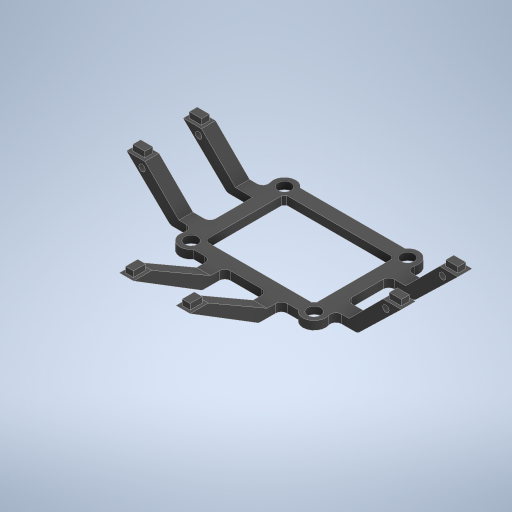
# Autodesk Inventor part: BasePlate
Saved by Autodesk Inventor 2024.2 (Build 282272000, 272)
## iProperties
Created: 2024-04-02
Part Number: BasePlate
Material: Generic
Document SubType Name: Modeling
Designer: ringl
Density: 1 g/cm^3
Appearance: Default(1)
Author: ringl
Autodesk Inventor part; units mm, degrees
sketch "Sketch1" plane through (0, 0, 0) normal (0, 1, 0) x (-1, 0, 0)
  circle A0 centre (0, 0) radius 2.35
  circle A1 centre (-43.5, 0) radius 2.35
  circle A2 centre (0, 33) radius 2.35
  circle A3 centre (-43.5, 33) radius 2.35
  line L0 (-3.2369, 30.65) -> (-40.2631, 30.65)
  line L1 (-40.2631, 35.35) -> (-3.2369, 35.35)
  line L2 (2.35, 29.7631) -> (2.35, 3.2369)
  line L3 (-2.35, 3.2369) -> (-2.35, 29.7631)
  line L4 (-3.2369, -2.35) -> (-40.2631, -2.35)
  line L5 (-40.2631, 2.35) -> (-3.2369, 2.35)
  arc A4 (-3.2369, -2.35) -> (2.35, 3.2369) centre (0, 0) ccw
  arc A5 (-2.35, 3.2369) -> (-3.2369, 2.35) centre (0, 0) ccw
  arc A6 (2.35, 29.7631) -> (-3.2369, 35.35) centre (0, 33) ccw
  arc A7 (-3.2369, 30.65) -> (-2.35, 29.7631) centre (0, 33) ccw
  line L6 (-41.15, 3.2369) -> (-41.15, 29.7631)
  line L7 (-45.85, 29.7631) -> (-45.85, 3.2369)
  arc A8 (-40.2631, 35.35) -> (-45.85, 29.7631) centre (-43.5, 33) ccw
  arc A9 (-41.15, 29.7631) -> (-40.2631, 30.65) centre (-43.5, 33) ccw
  arc A10 (-45.85, 3.2369) -> (-40.2631, -2.35) centre (-43.5, 0) ccw
  arc A11 (-40.2631, 2.35) -> (-41.15, 3.2369) centre (-43.5, 0) ccw
  dimension "d0" = 4.7
  dimension "d2" = 4.7
  dimension "d4" = 4.7
  dimension "d6" = 4.7
  dimension "d8" = 4
  dimension "d9" = 4
  dimension "d10" = 4
  dimension "d11" = 4
  dimension "d12" = 4
  dimension "d13" = 4
  dimension "d14" = 4
  dimension "d15" = 4
  dimension "d16" = 33
  dimension "d17" = 4.7
  dimension "d18" = 4.7
  dimension "d19" = 4.7
  dimension "d20" = 4.7
  dimension "d21" = 2.35
  dimension "d22" = 2.35
  dimension "d23" = 2.35
  dimension "d24" = 2.35
  dimension "d25" = 43.5
  constraints: 16 end point, 16 point on circle, 12 centre point, 5 coincident, 4 parallel, 2 horizontal, 2 horizontal alignment, 2 vertical alignment, 1 perpendicular, 1 vertical
  measures "d0" diameter of A0
  measures "d2" diameter of A1
  measures "d4" diameter of A2
  measures "d6" diameter of A3
  measures "d8" radius of A8
  measures "d9" radius of A6
  measures "d10" radius of A4
  measures "d11" radius of A10
  measures "d12" radius of A11
  measures "d13" radius of A9
  measures "d14" radius of A7
  measures "d15" radius of A5
  measures "d16" distance of A2.centre point (0, 0)
  measures "d17" distance between parallel lines of L1 L0
  measures "d18" distance between parallel lines of L7 L6
  measures "d19" distance between parallel lines of L4 L5
  measures "d20" distance between parallel lines of L2 L3
  measures "d21" distance from line of L0 A2.centre
  measures "d22" distance from line of A2.centre L3
  measures "d23" distance from line of L6 A3.centre
  measures "d24" distance from line of A1.centre L5
  measures "d25" distance of A1.centre point (0, 0)
extrude "Extrusion1" add sketch "Sketch1" along normal blind 3
chamfer "Chamfer1" distance 0.5 angle 45 4 edges at (2.35, 0, 33) (45.85, 0, 33) (45.85, 0, 0) (2.35, 0, 0)
ref_plane "Work Plane2" through (0, 0, 4) normal (0, 0, 1) x (1, 0, 0)
sketch "Sketch2" plane through (0, 0, 4) normal (0, 0, 1) x (1, 0, 0)
  line L0 (45.85, 0) -> (45.85, 3) projected
  line L1 (45.85, 0) -> (45.85, 3)
  line L2 (70.35, 15) -> (63.85, 15)
  line L3 (45.85, 0) -> (54.85, 0)
  line L4 (54.85, 0) -> (70.35, 15)
  line L5 (45.85, 3) -> (51.85, 3)
  line L6 (51.85, 3) -> (63.85, 15)
  point P0 (0, 0)
  point P1 (45.35, 2.077)
  point P2 (67.1, 15)
  dimension "d49" = 6.5
  dimension "d61" = 9
  dimension "d91" = 6
  dimension "d93" = 45
  dimension "d94" = 15
  constraints: 12 end point, 3 horizontal, 1 midpoint, 1 vertical
  measures "d49" distance of L2.start L2.end
  measures "d61" distance of L0.start L3.end
  measures "d91" distance of L0.end L5.end
  measures "d93" angle of L5 L6
  measures "d94" distance from line of point (67.1, 15) L3
extrude "Extrusion2" add sketch "Sketch2" along normal blind 5
ref_plane "Work Plane4" through (21.75, 0, 0) normal (1, 0, 0) x (0, 1, 0)
ref_plane "Work Plane5" through (0, 0, 16.5) normal (0, 0, 1) x (1, 0, 0)
mirror "Mirror1" about plane through (21.75, 0, 0) normal (1, 0, 0) of "Extrusion2"
mirror "Mirror2" about plane through (0, 0, 16.5) normal (0, 0, 1) of "Extrusion2", "Mirror1"
ref_plane "Work Plane6" through (9.25, 0, 0) normal (1, 0, 0) x (0, 1, 0)
sketch "Sketch7" plane through (9.25, 0, 0) normal (1, 0, 0) x (0, 1, 0)
  line L0 (0, 35.35) -> (3, 35.35) projected
  line L1 (0, 35.35) -> (0, 43.35)
  line L2 (0, 43.35) -> (15, 67.6346)
  line L3 (15, 67.6346) -> (15, 61.1346)
  line L4 (3, 35.35) -> (0, 35.35)
  line L5 (3, 35.35) -> (3, 40.35)
  line L6 (3, 29.7631) -> (3, 37) projected
  line L7 (3, 40.35) -> (15, 61.1346)
  point P0 (0, 0)
  point P1 (15, 64.3846)
  dimension "d72" = 8
  dimension "d73" = 6.5
  dimension "d95" = 15
  dimension "d98" = 5
  dimension "d99" = 30
  constraints: 12 end point, 1 collinear, 1 midpoint, 1 parallel, 1 perpendicular, 1 vertical
  measures "d72" distance of L0.start L1.end
  measures "d73" distance of L2.end L3.end
  measures "d95" distance from line of point (15, 64.385) L1
  measures "d98" distance of L0.end L5.end
  measures "d99" angle of L5 L7
extrude "Extrusion5" add sketch "Sketch7" along normal blind 5
mirror "Mirror5" about plane through (21.75, 0, 0) normal (1, 0, 0) of "Extrusion5"
sketch "Sketch5" plane through (63.85, 15, 4) normal (0, 1, 0) x (1, 0, 0)
  line L0 (5.4, -23.9) -> (1.1, -23.9)
  line L1 (1.1, -23.9) -> (1.1, -21.1)
  line L2 (1.1, -21.1) -> (5.4, -21.1)
  line L3 (5.4, -21.1) -> (5.4, -23.9)
  line L4 (6.5, -25) -> (6.5, -20) projected
  line L5 (6.5, -20) -> (0, -20) projected
  point P0 (-63.85, 4)
  dimension "d62" = 4.3
  dimension "d63" = 2.8
  dimension "d64" = 1.1
  dimension "d65" = 1.1
  constraints: 8 end point, 2 parallel, 1 horizontal, 1 perpendicular
  measures "d62" distance of L1.end L2.end
  measures "d63" distance of L0.end L1.end
  measures "d64" distance between parallel lines of L4 L3
  measures "d65" distance between parallel lines of L5 L2
extrude "Extrusion4" add sketch "Sketch5" along normal blind 2
mirror "Mirror3" about plane through (21.75, 0, 0) normal (1, 0, 0) of "Extrusion4"
mirror "Mirror4" about plane through (0, 0, 16.5) normal (0, 0, 1) of "Extrusion4", "Mirror3"
sketch "Sketch8" plane through (9.25, 15, 67.6346) normal (0, 1, 0) x (1, 0, 0)
  line L0 (1.1, 1.1) -> (3.9, 1.1)
  line L1 (3.9, 1.1) -> (3.9, 5.4)
  line L2 (3.9, 5.4) -> (1.1, 5.4)
  line L3 (1.1, 5.4) -> (1.1, 1.1)
  line L4 (21.1, 1.1) -> (23.9, 1.1)
  line L5 (23.9, 1.1) -> (23.9, 5.4)
  line L6 (23.9, 5.4) -> (21.1, 5.4)
  line L7 (21.1, 5.4) -> (21.1, 1.1)
  line L8 (25, 0) -> (20, 0) projected
  line L9 (25, 6.5) -> (25, 0) projected
  line L10 (5, 6.5) -> (5, 0) projected
  line L11 (0, 0) -> (5, 0) projected
  point P0 (-9.25, 67.6346)
  dimension "d78" = 2.8
  dimension "d79" = 4.3
  dimension "d80" = 2.8
  dimension "d81" = 4.3
  dimension "d82" = 1.1
  dimension "d83" = 1.1
  dimension "d84" = 1.1
  dimension "d85" = 1.1
  constraints: 16 end point, 4 parallel, 2 horizontal, 2 perpendicular
  measures "d78" distance of L2.end L1.end
  measures "d79" distance of L1.end L0.end
  measures "d80" distance of L6.end L5.end
  measures "d81" distance of L5.end L4.end
  measures "d82" distance between parallel lines of L8 L4
  measures "d83" distance between parallel lines of L9 L5
  measures "d84" distance between parallel lines of L10 L1
  measures "d85" distance between parallel lines of L11 L0
extrude "Extrusion6" add sketch "Sketch8" along normal blind 2
fillet "Fillet1" radius 2 15 edges at (-2.35, 1.5, 29.7631) (-2.35, 1.5, 29) (-2.35, 1.5, 24) (-2.35, 1.5, 4) (-2.35, 1.5, 3.2369) (45.85, 1.5, 3.2369) (45.85, 1.5, 4) (45.85, 1.5, 24) (45.85, 1.5, 9) (45.85, 1.5, 29.7631) (45.85, 1.5, 29) (34.25, 1.5, 35.35) (14.25, 1.5, 35.35) (29.25, 1.5, 35.35) (9.25, 1.5, 35.35)
fillet "Fillet2" radius 2 6 edges at (11.75, 0, 43.35) (31.75, 0, 43.35) (54.85, 0, 26.5) (54.85, 0, 6.5) (-11.35, 0, 26.5) (-11.35, 0, 6.5)
sketch "Sketch11" plane through (0, 0, 4) normal (0, 0, -1) x (-1, 0, 0)
  circle A0 centre (-64.85, 12.5) radius 1.15
  line L0 (-70.35, 15) -> (-63.85, 15) projected
  circle A1 centre (21.35, 12.5) radius 1.15
  line L1 (26.85, 15) -> (20.35, 15) projected
  point P0 (0, 0)
  point P1 (23.6, 15)
  dimension "d105" = 2.3
  dimension "d106" = 2.5
  dimension "d107" = 5.5
  dimension "d108" = 2.3
  dimension "d109" = 2.5
  dimension "d110" = 5.5
  constraints: 2 centre point, 1 midpoint
  measures "d105" diameter of A0
  measures "d106" distance from line of L0 A0.centre
  measures "d107" horizontal distance of L0.start A0.centre
  measures "d108" diameter of A1
  measures "d109" vertical distance of point (23.6, 15) A1.centre
  measures "d110" horizontal distance of L1.start A1.centre
extrude "Extrusion8" cut sketch "Sketch11" against normal through all
body "Solid1"
